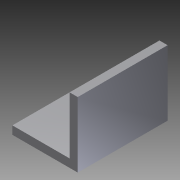
# Autodesk Inventor part: L frame short
Saved by Autodesk Inventor 2012 (Build 160160000, 160)
## iProperties
Created: 2012-08-16
Part Number: L frame short
Material: Default
Document SubType Name: Modeling
Designer: Bryce
Density: 1 g/cm^3
Author: Bryce
Autodesk Inventor part; units mm, degrees
ref_plane "YZ Plane" through (0, 0, 0) normal (1, 0, 0) x (0, 1, 0)
ref_plane "XZ Plane" through (0, 0, 0) normal (0, 1, 0) x (-1, 0, 0)
ref_plane "XY Plane" through (0, 0, 0) normal (0, 0, 1) x (1, 0, 0)
sketch "Sketch1" plane through (0, 0, 0) normal (0, 0, 1) x (1, 0, 0)
  line L0 (-25.4, 0) -> (0, 0)
  line L1 (0, 0) -> (0, 25.4)
  line L2 (0, 25.4) -> (-3.175, 25.4)
  line L3 (-3.175, 25.4) -> (-3.175, 3.175)
  line L4 (-3.175, 3.175) -> (-25.4, 3.175)
  line L5 (-25.4, 3.175) -> (-25.4, 0)
  dimension "d0" = 3.175
  dimension "d1" = 3.175
  dimension "d2" = 25.4
  dimension "d3" = 25.4
  constraints: 12 end point, 4 parallel, 1 horizontal, 1 perpendicular
  measures "d0" distance between parallel lines of L0 L4
  measures "d1" distance between parallel lines of L3 L1
  measures "d2" distance of L0.end L1.end
  measures "d3" distance of L0.start L0.end
extrude "Extrusion1" add sketch "Sketch1" along normal blind 34.925
body "Solid1"
